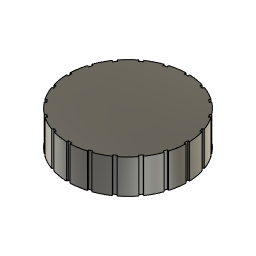
3DKNOB v3 (Autodesk Fusion 360 design; units mm, degrees)
Autodesk Fusion 360 part; units mm, degrees
sketch "Sketch1" plane through (0, 0, 0) normal (0, 0, 1) x (1, 0, 0)
  line L0 (0, 0) -> (124, 0)
  line L1 (124, 0) -> (124, 124)
  line L2 (124, 124) -> (0, 124)
  line L3 (0, 124) -> (0, 0)
  dimension "d1" = 124
  dimension "d2" = 124
  constraint horizontal L0
  constraint vertical L1
  constraint horizontal L2
  constraint vertical L3
  constraint coincident L0.start L3.end
  measures "d1" distance of L0.start L0.end
  measures "d2" distance of L0.start L2.end
sketch "Sketch3" plane through (0, 0, 5) normal (0, 0, 1) x (-1, 0, 0)
  line L0 (0, -124) -> (0, 0)
  line L1 (0, 0) -> (-124, 0)
  line L2 (-124, 0) -> (-124, -124)
  line L3 (-124, -124) -> (0, -124)
  line L4 (0, 0) -> (-124, 0)
  line L5 (-124, 0) -> (-124, -124)
  line L6 (-124, -124) -> (0, -124)
  line L7 (0, -124) -> (0, 0)
  line L8 (0, -124) -> (-124, -124)
  line L9 (-124, -124) -> (-124, 0)
  line L10 (-124, 0) -> (0, 0)
  line L11 (0, 0) -> (0, -124)
  line L12 (0, -124) -> (-7, -124)
  line L13 (-7, -124) -> (-7, -117)
  line L14 (-7, -117) -> (0, -117)
  line L15 (0, -117) -> (0, -124)
  line L16 (-7, -117) -> (-117, -117)
  line L17 (-117, -117) -> (-117, -7)
  line L18 (-117, -7) -> (-7, -7)
  line L19 (-7, -7) -> (-7, -117)
  line L20 (-7, -117) -> (-12, -117)
  line L21 (-12, -117) -> (-12, -112)
  line L22 (-12, -112) -> (-7, -112)
  line L23 (-7, -112) -> (-7, -117)
  line L24 (-12, -112) -> (-112, -112)
  line L25 (-112, -112) -> (-112, -12)
  line L26 (-112, -12) -> (-12, -12)
  line L27 (-12, -12) -> (-12, -112)
  dimension "d5" = 7
  dimension "d6" = 7
  dimension "d7" = 110
  dimension "d8" = 110
  dimension "d9" = 5
  dimension "d10" = 5
  dimension "d11" = 100
  dimension "d12" = 100
  constraint horizontal L4
  constraint vertical L5
  constraint horizontal L6
  constraint vertical L7
  constraint coincident L2.end L3.start
  constraint coincident L0.end L1.start
  constraint horizontal L8
  constraint vertical L9
  constraint horizontal L10
  constraint vertical L11
  constraint coincident L1.end L2.start
  constraint coincident L0.start L3.end
  constraint horizontal L12
  constraint vertical L13
  constraint horizontal L14
  constraint vertical L15
  constraint horizontal L16
  constraint vertical L17
  constraint horizontal L18
  constraint vertical L19
  constraint horizontal L20
  constraint vertical L21
  constraint horizontal L22
  constraint vertical L23
  constraint horizontal L24
  constraint vertical L25
  constraint horizontal L26
  constraint vertical L27
  measures "d5" distance of L0.start L12.end
  measures "d6" distance of L0.start L14.end
  measures "d7" distance of L13.end L16.end
  measures "d8" distance of L13.end L18.end
  measures "d9" distance of L13.end L20.end
  measures "d10" distance of L13.end L22.end
  measures "d11" distance of L21.end L24.end
  measures "d12" distance of L21.end L26.end
sketch "Sketch4" plane through (0, 12, 0) normal (0, -1, 0) x (1, 0, 0)
  line L0 (12, 5) -> (112, 5)
  line L1 (112, 5) -> (112, 10)
  line L2 (112, 10) -> (12, 10)
  line L3 (12, 10) -> (12, 5)
  line L4 (12, 5) -> (112, 5)
  line L5 (112, 5) -> (112, 75)
  line L6 (112, 75) -> (12, 75)
  line L7 (12, 75) -> (12, 5)
  line L8 (112, 5) -> (112, 22.5)
  line L9 (112, 22.5) -> (107, 22.5)
  line L10 (107, 22.5) -> (107, 17.5)
  line L11 (107, 17.5) -> (112, 17.5)
  line L12 (112, 17.5) -> (112, 22.5)
  line L13 (112, 22.5) -> (107, 22.5)
  line L14 (107, 22.5) -> (107, 27.5)
  line L15 (107, 27.5) -> (112, 27.5)
  line L16 (112, 27.5) -> (112, 22.5)
  line L17 (112, 75) -> (112, 57.5)
  line L18 (112, 57.5) -> (107, 57.5)
  line L19 (107, 57.5) -> (107, 62.5)
  line L20 (107, 62.5) -> (112, 62.5)
  line L21 (112, 62.5) -> (112, 57.5)
  line L22 (112, 57.5) -> (107, 57.5)
  line L23 (107, 57.5) -> (107, 52.5)
  line L24 (107, 52.5) -> (112, 52.5)
  line L25 (112, 52.5) -> (112, 57.5)
  line L26 (12, 75) -> (12, 57.5)
  line L27 (12, 57.5) -> (17, 57.5)
  line L28 (17, 57.5) -> (17, 62.5)
  line L29 (17, 62.5) -> (12, 62.5)
  line L30 (12, 62.5) -> (12, 57.5)
  line L31 (12, 57.5) -> (17, 57.5)
  line L32 (17, 57.5) -> (17, 52.5)
  line L33 (17, 52.5) -> (12, 52.5)
  line L34 (12, 52.5) -> (12, 57.5)
  line L35 (12, 5) -> (12, 22.5)
  line L36 (12, 22.5) -> (17, 22.5)
  line L37 (17, 22.5) -> (17, 27.5)
  line L38 (17, 27.5) -> (12, 27.5)
  line L39 (12, 27.5) -> (12, 22.5)
  line L40 (12, 22.5) -> (17, 22.5)
  line L41 (17, 22.5) -> (17, 17.5)
  line L42 (17, 17.5) -> (12, 17.5)
  line L43 (12, 17.5) -> (12, 22.5)
  line L44 (12, 62.5) -> (7, 62.5)
  line L45 (7, 62.5) -> (7, 52.5)
  line L46 (7, 52.5) -> (12, 52.5)
  line L47 (12, 52.5) -> (12, 62.5)
  line L48 (12, 27.5) -> (7, 27.5)
  line L49 (7, 27.5) -> (7, 17.5)
  line L50 (7, 17.5) -> (12, 17.5)
  line L51 (12, 17.5) -> (12, 27.5)
  line L52 (112, 62.5) -> (117, 62.5)
  line L53 (117, 62.5) -> (117, 52.5)
  line L54 (117, 52.5) -> (112, 52.5)
  line L55 (112, 52.5) -> (112, 62.5)
  line L56 (112, 27.5) -> (117, 27.5)
  line L57 (117, 27.5) -> (117, 17.5)
  line L58 (117, 17.5) -> (112, 17.5)
  line L59 (112, 17.5) -> (112, 27.5)
  dimension "d15" = 100
  dimension "d16" = 70
  dimension "d17" = 17.5
  dimension "d18" = 5
  dimension "d19" = 5
  dimension "d20" = 5
  dimension "d21" = 5
  dimension "d22" = 17.5
  dimension "d23" = 5
  dimension "d24" = 5
  dimension "d25" = 5
  dimension "d26" = 5
  dimension "d27" = 17.5
  dimension "d28" = 5
  dimension "d29" = 5
  dimension "d30" = 5
  dimension "d31" = 5
  dimension "d32" = 17.5
  dimension "d33" = 5
  dimension "d34" = 5
  dimension "d35" = 5
  dimension "d36" = 5
  dimension "d37" = 5
  dimension "d38" = 10
  dimension "d39" = 5
  dimension "d40" = 10
  dimension "d41" = 5
  dimension "d42" = 10
  dimension "d43" = 5
  dimension "d44" = 10
  constraint horizontal L4
  constraint vertical L5
  constraint horizontal L6
  constraint vertical L7
  constraint coincident L0.start L3.end
  constraint coincident L0.end L1.start
  constraint perpendicular L4 L8
  constraint horizontal L9
  constraint vertical L10
  constraint horizontal L11
  constraint vertical L12
  constraint horizontal L13
  constraint vertical L14
  constraint horizontal L15
  constraint vertical L16
  constraint perpendicular L6 L17
  constraint horizontal L18
  constraint vertical L19
  constraint horizontal L20
  constraint vertical L21
  constraint horizontal L22
  constraint vertical L23
  constraint horizontal L24
  constraint vertical L25
  constraint perpendicular L6 L26
  constraint horizontal L27
  constraint vertical L28
  constraint horizontal L29
  constraint vertical L30
  constraint horizontal L31
  constraint vertical L32
  constraint horizontal L33
  constraint vertical L34
  constraint perpendicular L4 L35
  constraint horizontal L36
  constraint vertical L37
  constraint horizontal L38
  constraint vertical L39
  constraint horizontal L40
  constraint vertical L41
  constraint horizontal L42
  constraint vertical L43
  constraint horizontal L44
  constraint vertical L45
  constraint horizontal L46
  constraint vertical L47
  constraint horizontal L48
  constraint vertical L49
  constraint horizontal L50
  constraint vertical L51
  constraint horizontal L52
  constraint vertical L53
  constraint horizontal L54
  constraint vertical L55
  constraint horizontal L56
  constraint vertical L57
  constraint horizontal L58
  constraint vertical L59
  measures "d15" distance of L0.start L0.end
  measures "d16" distance of L0.start L6.end
  measures "d17" distance of L0.end L8.end
  measures "d18" distance of L8.end L9.end
  measures "d19" distance of L8.end L11.end
  measures "d20" distance of L8.end L9.end
  measures "d21" distance of L8.end L15.end
  measures "d22" distance of L5.end L17.end
  measures "d23" distance of L17.end L18.end
  measures "d24" distance of L17.end L20.end
  measures "d25" distance of L17.end L18.end
  measures "d26" distance of L17.end L24.end
  measures "d27" distance of L6.end L26.end
  measures "d28" distance of L26.end L27.end
  measures "d29" distance of L26.end L29.end
  measures "d30" distance of L26.end L27.end
  measures "d31" distance of L26.end L33.end
  measures "d32" distance of L0.start L35.end
  measures "d33" distance of L35.end L36.end
  measures "d34" distance of L35.end L38.end
  measures "d35" distance of L35.end L36.end
  measures "d36" distance of L35.end L42.end
  measures "d37" distance of L29.end L44.end
  measures "d38" distance of L29.end L33.end
  measures "d39" distance of L38.end L48.end
  measures "d40" distance of L38.end L42.end
  measures "d41" distance of L20.end L52.end
  measures "d42" distance of L20.end L24.end
  measures "d43" distance of L15.end L56.end
  measures "d44" distance of L15.end L11.end
sketch "Sketch5" plane through (0, 112, 0) normal (0, 1, 0) x (-1, 0, 0)
  line L0 (-112, 5) -> (-12, 5)
  line L1 (-12, 5) -> (-12, 10)
  line L2 (-12, 10) -> (-112, 10)
  line L3 (-112, 10) -> (-112, 5)
  line L4 (-112, 5) -> (-12, 5)
  line L5 (-12, 5) -> (-12, 35)
  line L6 (-12, 35) -> (-112, 35)
  line L7 (-112, 35) -> (-112, 5)
  line L8 (-12, 35) -> (-12, 20)
  line L9 (-12, 20) -> (-7, 20)
  line L10 (-7, 20) -> (-7, 25)
  line L11 (-7, 25) -> (-12, 25)
  line L12 (-12, 25) -> (-12, 20)
  line L13 (-12, 20) -> (-7, 20)
  line L14 (-7, 20) -> (-7, 15)
  line L15 (-7, 15) -> (-12, 15)
  line L16 (-12, 15) -> (-12, 20)
  line L17 (-112, 20) -> (-117, 20)
  line L18 (-117, 20) -> (-117, 25)
  line L19 (-117, 25) -> (-112, 25)
  line L20 (-112, 25) -> (-112, 20)
  line L21 (-112, 20) -> (-117, 20)
  line L22 (-117, 20) -> (-117, 15)
  line L23 (-117, 15) -> (-112, 15)
  line L24 (-112, 15) -> (-112, 20)
  dimension "d47" = 100
  dimension "d48" = 30
  dimension "d49" = 15
  dimension "d50" = 5
  dimension "d51" = 5
  dimension "d52" = 5
  dimension "d53" = 5
  dimension "d54" = 5
  dimension "d55" = 5
  dimension "d56" = 5
  dimension "d57" = 5
  constraint horizontal L4
  constraint vertical L5
  constraint horizontal L6
  constraint vertical L7
  constraint coincident L0.start L3.end
  constraint perpendicular L6 L8
  constraint horizontal L9
  constraint vertical L10
  constraint horizontal L11
  constraint vertical L12
  constraint horizontal L13
  constraint vertical L14
  constraint horizontal L15
  constraint vertical L16
  constraint horizontal L17
  constraint vertical L18
  constraint horizontal L19
  constraint vertical L20
  constraint midpoint L7 L17.start
  constraint horizontal L21
  constraint vertical L22
  constraint horizontal L23
  constraint vertical L24
  measures "d47" distance of L0.start L0.end
  measures "d48" distance of L0.start L6.end
  measures "d49" distance of L5.end L8.end
  measures "d50" distance of L8.end L9.end
  measures "d51" distance of L8.end L11.end
  measures "d52" distance of L8.end L9.end
  measures "d53" distance of L8.end L15.end
  measures "d54" distance of L17.start L17.end
  measures "d55" distance of L17.start L19.end
  measures "d56" distance of L17.start L17.end
  measures "d57" distance of L17.start L23.end
sketch "Sketch6" plane through (12, 0, 0) normal (-1, 0, 0) x (0, -1, 0)
  line L0 (-112, 5) -> (-12, 5)
  line L1 (-12, 5) -> (-12, 10)
  line L2 (-12, 10) -> (-112, 10)
  line L3 (-112, 10) -> (-112, 5)
  line L4 (-117, 5) -> (-7, 5)
  line L5 (-7, 5) -> (-7, 35)
  line L6 (-7, 35) -> (-117, 35)
  line L7 (-117, 35) -> (-117, 5)
  line L8 (-117, 35) -> (-7, 75)
  line L9 (-7, 75) -> (-7, 35)
  line L10 (-7, 75) -> (-7, 62.5)
  line L11 (-7, 62.5) -> (-12, 62.5)
  line L12 (-12, 62.5) -> (-12, 52.5)
  line L13 (-12, 52.5) -> (-7, 52.5)
  line L14 (-7, 52.5) -> (-7, 62.5)
  line L15 (-7, 5) -> (-7, 17.5)
  line L16 (-7, 17.5) -> (-12, 17.5)
  line L17 (-12, 17.5) -> (-12, 27.5)
  line L18 (-12, 27.5) -> (-7, 27.5)
  line L19 (-7, 27.5) -> (-7, 17.5)
  line L20 (-117, 5) -> (-117, 15)
  line L21 (-117, 15) -> (-112, 15)
  line L22 (-112, 15) -> (-112, 25)
  line L23 (-112, 25) -> (-117, 25)
  line L24 (-117, 25) -> (-117, 15)
  dimension "d60" = 110
  dimension "d61" = 30
  dimension "d62" = 12.5
  dimension "d63" = 5
  dimension "d64" = 10
  dimension "d65" = 12.5
  dimension "d66" = 5
  dimension "d67" = 10
  dimension "d68" = 10
  dimension "d69" = 5
  dimension "d70" = 10
  constraint horizontal L4
  constraint vertical L5
  constraint horizontal L6
  constraint vertical L7
  constraint parallel L9 L10
  constraint vertical L12
  constraint perpendicular L11 L12
  constraint horizontal L13
  constraint parallel L12 L14
  constraint perpendicular L6 L15
  constraint vertical L17
  constraint perpendicular L16 L17
  constraint horizontal L18
  constraint parallel L17 L19
  constraint perpendicular L4 L20
  constraint horizontal L21
  constraint vertical L22
  constraint horizontal L23
  constraint vertical L24
  measures "d60" distance of L4.start L4.end
  measures "d61" distance of L4.start L6.end
  measures "d62" distance of L8.end L10.end
  measures "d63" distance of L10.end L11.end
  measures "d64" distance of L10.end L13.end
  measures "d65" distance of L4.end L15.end
  measures "d66" distance of L15.end L16.end
  measures "d67" distance of L15.end L18.end
  measures "d68" distance of L4.start L20.end
  measures "d69" distance of L20.end L21.end
  measures "d70" distance of L20.end L23.end
sketch "Sketch7" plane through (112, 0, 0) normal (1, 0, 0) x (0, 1, 0)
  line L0 (12, 5) -> (112, 5)
  line L1 (112, 5) -> (112, 10)
  line L2 (112, 10) -> (12, 10)
  line L3 (12, 10) -> (12, 5)
  line L4 (12, 5) -> (117, 5)
  line L5 (117, 5) -> (117, 35)
  line L6 (117, 35) -> (12, 35)
  line L7 (12, 35) -> (12, 5)
  line L8 (12, 5) -> (7, 5)
  line L9 (7, 5) -> (7, 35)
  line L10 (7, 35) -> (12, 35)
  line L11 (12, 35) -> (12, 5)
  line L12 (7, 35) -> (7, 75)
  line L13 (7, 75) -> (117, 35)
  line L14 (7, 75) -> (7, 62.5)
  line L15 (7, 62.5) -> (12, 62.5)
  line L16 (12, 62.5) -> (12, 52.5)
  line L17 (12, 52.5) -> (7, 52.5)
  line L18 (7, 52.5) -> (7, 62.5)
  line L19 (7, 5) -> (7, 17.5)
  line L20 (7, 17.5) -> (12, 17.5)
  line L21 (12, 17.5) -> (12, 27.5)
  line L22 (12, 27.5) -> (7, 27.5)
  line L23 (7, 27.5) -> (7, 17.5)
  line L24 (117, 20) -> (112, 20)
  line L25 (112, 20) -> (112, 25)
  line L26 (112, 25) -> (117, 25)
  line L27 (117, 25) -> (117, 20)
  line L28 (117, 20) -> (112, 20)
  line L29 (112, 20) -> (112, 15)
  line L30 (112, 15) -> (117, 15)
  line L31 (117, 15) -> (117, 20)
  dimension "d73" = 105
  dimension "d74" = 30
  dimension "d75" = 12.5
  dimension "d76" = 5
  dimension "d77" = 10
  dimension "d78" = 12.5
  dimension "d79" = 5
  dimension "d80" = 10
  dimension "d81" = 5
  dimension "d82" = 5
  dimension "d83" = 5
  dimension "d84" = 5
  constraint horizontal L4
  constraint vertical L5
  constraint horizontal L6
  constraint vertical L7
  constraint coincident L0.start L3.end
  constraint horizontal L8
  constraint vertical L9
  constraint horizontal L10
  constraint vertical L11
  constraint perpendicular L10 L12
  constraint perpendicular L6 L14
  constraint horizontal L15
  constraint vertical L16
  constraint horizontal L17
  constraint vertical L18
  constraint perpendicular L8 L19
  constraint horizontal L20
  constraint vertical L21
  constraint horizontal L22
  constraint vertical L23
  constraint horizontal L24
  constraint vertical L25
  constraint horizontal L26
  constraint vertical L27
  constraint midpoint L5 L24.start
  constraint horizontal L28
  constraint vertical L29
  constraint horizontal L30
  constraint vertical L31
  measures "d73" distance of L0.start L4.end
  measures "d74" distance of L0.start L6.end
  measures "d75" distance of L12.end L14.end
  measures "d76" distance of L14.end L15.end
  measures "d77" distance of L14.end L17.end
  measures "d78" distance of L8.end L19.end
  measures "d79" distance of L19.end L20.end
  measures "d80" distance of L19.end L22.end
  measures "d81" distance of L24.start L24.end
  measures "d82" distance of L24.start L26.end
  measures "d83" distance of L24.start L24.end
  measures "d84" distance of L24.start L30.end
sketch "Sketch8" plane through (112, 0, 0) normal (1, 0, 0) x (0, 1, 0)
  line L0 (12, 62.5) -> (12, 75)
  line L1 (12, 75) -> (7, 75)
  line L2 (7, 75) -> (7, 62.5)
  line L3 (7, 62.5) -> (12, 62.5)
  line L4 (12, 75) -> (12, 73.2)
  line L5 (12, 75) -> (7, 75)
  line L6 (7, 75) -> (12, 73.2)
  constraint coincident L0.end L1.start
  constraint coincident L0 L4.end
  constraint perpendicular L1 L4
  constraint coincident L1.end L2.start
sketch "Sketch9" plane through (0, 24.9051, 68.4891) normal (0, 0.341743, 0.939793) x (-1, 0, 0)
  line L0 (-12, 19.0522) -> (-12, -97.9948)
  line L1 (-12, -97.9948) -> (-7, -97.9948)
  line L2 (-7, -97.9948) -> (-7, 19.0522)
  line L3 (-7, 19.0522) -> (-12, 19.0522)
  line L4 (-112, 13) -> (-12, 13)
  line L5 (-12, 13) -> (-12, -93.0081)
  line L6 (-12, -93.0081) -> (-112, -93.0081)
  line L7 (-112, -93.0081) -> (-112, 13)
  constraint horizontal L4
  constraint vertical L5
  constraint horizontal L6
  constraint vertical L7
  constraint coincident L0 L5.end
sketch "Sketch10" plane through (0, 24.9051, 68.4891) normal (0, 0.341743, 0.939793) x (-1, 0, 0)
  line L0 (-112, -93.0081) -> (-12, -93.0081)
  line L1 (-12, -93.0081) -> (-12, 13)
  line L2 (-12, 13) -> (-112, 13)
  line L3 (-112, 13) -> (-112, -93.0081)
  line L4 (-117, -98) -> (-7, -98)
  line L5 (-7, -98) -> (-7, 19.05)
  line L6 (-7, 19.05) -> (-117, 19.05)
  line L7 (-117, 19.05) -> (-117, -98)
  constraint horizontal L4
  constraint vertical L5
  constraint horizontal L6
  constraint vertical L7
sketch "Sketch11" plane through (117, 0, 0) normal (1, 0, 0) x (0, 1, 0)
  line L0 (7.002, 74.9993) -> (117.0049, 34.9982)
  line L1 (117.0049, 34.9982) -> (118.7136, 39.6972)
  line L2 (118.7136, 39.6972) -> (8.7108, 79.6982)
  line L3 (8.7108, 79.6982) -> (7.002, 74.9993)
  line L4 (117.0049, 34.9982) -> (117.0049, 40.3185)
  line L5 (118.7136, 39.6972) -> (117.0049, 34.9982)
  line L6 (118.7136, 39.6972) -> (117.0049, 40.3185)
  constraint coincident L0.end L1.start
  constraint coincident L2 L4.end
  constraint vertical L4
  constraint coincident L1.end L2.start
sketch "Sketch14" plane through (0, 26.6138, 73.188) normal (0, 0.341743, 0.939793) x (-1, 0, 0)
  line L0 (-117, -96.1818) -> (-7, -96.1818)
  line L1 (-7, -96.1818) -> (-7, 19.05)
  line L2 (-7, 19.05) -> (-117, 19.05)
  line L3 (-117, 19.05) -> (-117, -96.1818)
  circle A0 centre (-62, -38.5659) radius 35
  line L4 (-62, -38.5659) -> (-62, -3.5659)
  line L5 (-62, -3.5659) -> (-61, -3.5659)
  line L6 (-61, -3.5659) -> (-61, -4.5659)
  line L7 (-61, -4.5659) -> (-62, -4.5659)
  line L8 (-62, -4.5659) -> (-62, -3.5659)
  line L9 (-62, -3.5659) -> (-63, -3.5659)
  line L10 (-63, -3.5659) -> (-63, -4.5659)
  line L11 (-63, -4.5659) -> (-62, -4.5659)
  line L12 (-62, -4.5659) -> (-62, -3.5659)
  dimension "d105" = 70
  dimension "d106" = 1
  dimension "d107" = 1
  dimension "d108" = 1
  constraint coincident A0.centre L4.start
  constraint coincident A0 L4.end
  constraint vertical L4
  constraint horizontal L5
  constraint vertical L6
  constraint horizontal L7
  constraint vertical L8
  constraint horizontal L9
  constraint vertical L10
  constraint horizontal L11
  constraint vertical L12
  measures "d105" diameter of A0
  measures "d106" distance of L4.end L5.end
  measures "d107" distance of L4.end L7.end
  measures "d108" distance of L4.end L7.end
extrude "Extrude12" add sketch "Sketch14" along normal blind 20 contours A0 L6 L7 L10 L11
pattern_circular "C-Pattern1" count 20 over 360 about axis through (62, 69.6927, 78.8043) along (0, 0.341743, 0.939793) of 3 faces at (62.3333, 33.1831, 77.8929) (63, 34.8438, 84.3828) (61, 32.8743, 78.0052)
sketch "Sketch15" plane through (0, 26.6138, 73.188) normal (0, -0.341743, -0.939793) x (1, 0, 0)
  line L0 (52.1399, -4.9835) -> (52.4445, -5.921)
  line L1 (52.4445, -5.921) -> (50.5424, -6.539)
  line L2 (50.5424, -6.539) -> (50.2378, -5.6015)
  arc A0 (50.2378, -5.6015) -> (42.2449, -9.6741) centre (62, -38.5659) ccw
  line L3 (42.2449, -9.6741) -> (42.8243, -10.4715)
  line L4 (42.8243, -10.4715) -> (41.2063, -11.6471)
  line L5 (41.2063, -11.6471) -> (40.6269, -10.8497)
  arc A1 (40.6269, -10.8497) -> (34.2838, -17.1928) centre (62, -38.5659) ccw
  line L6 (34.2838, -17.1928) -> (35.0812, -17.7722)
  line L7 (35.0812, -17.7722) -> (33.9056, -19.3902)
  line L8 (33.9056, -19.3902) -> (33.1082, -18.8108)
  arc A2 (33.1082, -18.8108) -> (29.0356, -26.8037) centre (62, -38.5659) ccw
  line L9 (29.0356, -26.8037) -> (29.9731, -27.1083)
  line L10 (29.9731, -27.1083) -> (29.3551, -29.0104)
  line L11 (29.3551, -29.0104) -> (28.4176, -28.7058)
  arc A3 (28.4176, -28.7058) -> (27.0143, -37.5659) centre (62, -38.5659) ccw
  line L12 (27.0143, -37.5659) -> (28, -37.5659)
  line L13 (28, -37.5659) -> (28, -39.5659)
  line L14 (28, -39.5659) -> (27.0143, -39.5659)
  arc A4 (27.0143, -39.5659) -> (28.4176, -48.426) centre (62, -38.5659) ccw
  line L15 (28.4176, -48.426) -> (29.3551, -48.1214)
  line L16 (29.3551, -48.1214) -> (29.9731, -50.0235)
  line L17 (29.9731, -50.0235) -> (29.0356, -50.3281)
  arc A5 (29.0356, -50.3281) -> (33.1082, -58.321) centre (62, -38.5659) ccw
  line L18 (33.1082, -58.321) -> (33.9056, -57.7416)
  line L19 (33.9056, -57.7416) -> (35.0812, -59.3596)
  line L20 (35.0812, -59.3596) -> (34.2838, -59.939)
  arc A6 (34.2838, -59.939) -> (40.6269, -66.2822) centre (62, -38.5659) ccw
  line L21 (40.6269, -66.2822) -> (41.2063, -65.4847)
  line L22 (41.2063, -65.4847) -> (42.8243, -66.6603)
  line L23 (42.8243, -66.6603) -> (42.2449, -67.4577)
  arc A7 (42.2449, -67.4577) -> (50.2378, -71.5303) centre (62, -38.5659) ccw
  line L24 (50.2378, -71.5303) -> (50.5424, -70.5928)
  line L25 (50.5424, -70.5928) -> (52.4445, -71.2108)
  line L26 (52.4445, -71.2108) -> (52.1399, -72.1483)
  arc A8 (52.1399, -72.1483) -> (61, -73.5516) centre (62, -38.5659) ccw
  line L27 (61, -73.5516) -> (61, -72.5659)
  line L28 (61, -72.5659) -> (63, -72.5659)
  line L29 (63, -72.5659) -> (63, -73.5516)
  arc A9 (63, -73.5516) -> (71.8601, -72.1483) centre (62, -38.5659) ccw
  line L30 (71.8601, -72.1483) -> (71.5555, -71.2108)
  line L31 (71.5555, -71.2108) -> (73.4576, -70.5928)
  line L32 (73.4576, -70.5928) -> (73.7622, -71.5303)
  arc A10 (73.7622, -71.5303) -> (81.7551, -67.4577) centre (62, -38.5659) ccw
  line L33 (81.7551, -67.4577) -> (81.1757, -66.6603)
  line L34 (81.1757, -66.6603) -> (82.7937, -65.4847)
  line L35 (82.7937, -65.4847) -> (83.3731, -66.2822)
  arc A11 (83.3731, -66.2822) -> (89.7163, -59.939) centre (62, -38.5659) ccw
  line L36 (89.7163, -59.939) -> (88.9188, -59.3596)
  line L37 (88.9188, -59.3596) -> (90.0944, -57.7416)
  line L38 (90.0944, -57.7416) -> (90.8918, -58.321)
  arc A12 (90.8918, -58.321) -> (94.9644, -50.3281) centre (62, -38.5659) ccw
  line L39 (94.9644, -50.3281) -> (94.0269, -50.0235)
  line L40 (94.0269, -50.0235) -> (94.6449, -48.1214)
  line L41 (94.6449, -48.1214) -> (95.5824, -48.426)
  arc A13 (95.5824, -48.426) -> (96.9857, -39.5659) centre (62, -38.5659) ccw
  line L42 (96.9857, -39.5659) -> (96, -39.5659)
  line L43 (96, -39.5659) -> (96, -37.5659)
  line L44 (96, -37.5659) -> (96.9857, -37.5659)
  arc A14 (96.9857, -37.5659) -> (95.5824, -28.7058) centre (62, -38.5659) ccw
  line L45 (95.5824, -28.7058) -> (94.6449, -29.0104)
  line L46 (94.6449, -29.0104) -> (94.0269, -27.1083)
  line L47 (94.0269, -27.1083) -> (94.9644, -26.8037)
  arc A15 (94.9644, -26.8037) -> (90.8918, -18.8108) centre (62, -38.5659) ccw
  line L48 (90.8918, -18.8108) -> (90.0944, -19.3902)
  line L49 (90.0944, -19.3902) -> (88.9188, -17.7722)
  line L50 (88.9188, -17.7722) -> (89.7163, -17.1928)
  arc A16 (89.7163, -17.1928) -> (83.3731, -10.8497) centre (62, -38.5659) ccw
  line L51 (83.3731, -10.8497) -> (82.7937, -11.6471)
  line L52 (82.7937, -11.6471) -> (81.1757, -10.4715)
  line L53 (81.1757, -10.4715) -> (81.7551, -9.6741)
  arc A17 (81.7551, -9.6741) -> (73.7622, -5.6015) centre (62, -38.5659) ccw
  line L54 (73.7622, -5.6015) -> (73.4576, -6.539)
  line L55 (73.4576, -6.539) -> (71.5555, -5.921)
  line L56 (71.5555, -5.921) -> (71.8601, -4.9835)
  arc A18 (71.8601, -4.9835) -> (63, -3.5802) centre (62, -38.5659) ccw
  line L57 (63, -3.5802) -> (63, -4.5659)
  line L58 (63, -4.5659) -> (61, -4.5659)
  line L59 (61, -4.5659) -> (61, -3.5802)
  arc A19 (61, -3.5802) -> (52.1399, -4.9835) centre (62, -38.5659) ccw
  circle A20 centre (62, -38.5659) radius 3
  line L60 (62, -38.5659) -> (62, -38.1159)
  line L61 (62, -38.5659) -> (62, -39.0159)
  line L62 (62, -38.1159) -> (64.9661, -38.1159)
  line L63 (62, -39.0159) -> (64.9661, -39.0159)
  line L64 (62, -38.1159) -> (59.0339, -38.1159)
  line L65 (62, -39.0159) -> (59.0339, -39.0159)
  dimension "d115" = 6
  dimension "d116" = 0.45
  dimension "d117" = 0.45
  constraint concentric A0 A20
  constraint coincident A0.centre A1.centre
  constraint vertical L60
  constraint parallel L60 L61
  constraint coincident A20 L62.end
  constraint perpendicular L60 L62
  constraint coincident A20 L63.end
  constraint perpendicular L61 L63
  constraint coincident A20 L64.end
  constraint perpendicular L60 L64
  constraint coincident A20 L65.end
  constraint perpendicular L61 L65
  measures "d115" diameter of A20
  measures "d116" distance of A0.centre L60.end
  measures "d117" distance of A0.centre L61.end
extrude "Extrude13" cut sketch "Sketch15" against normal blind 10 contours A20 L62 L64 | A20 L63 L65
sketch "Sketch16" plane through (0, 24.9051, 68.4891) normal (0, -0.341743, -0.939793) x (1, 0, 0)
  line L0 (117, -98) -> (117, 19.05)
  line L1 (117, 19.05) -> (7, 19.05)
  line L2 (7, 19.05) -> (7, -98)
  line L3 (7, -98) -> (117, -98)
  circle A0 centre (62, -39.475) radius 4
  dimension "d120" = 8
  measures "d120" diameter of A0
sketch "Sketch17" plane through (0, 24.9051, 68.4891) normal (0, 0.341743, 0.939793) x (-1, 0, 0)
  line L0 (-112, -93.0081) -> (-12, -93.0081)
  line L1 (-12, -93.0081) -> (-12, 13)
  line L2 (-12, 13) -> (-112, 13)
  line L3 (-112, 13) -> (-112, -93.0081)
  circle A0 centre (-62, -39.474) radius 4
  dimension "d123" = 8
  measures "d123" diameter of A0
sketch "Sketch18" plane through (12, 0, 0) normal (-1, 0, 0) x (0, -1, 0)
  line L0 (-12.6878, 72.9317) -> (-112.3135, 36.7042)
  line L1 (-112.3135, 36.7042) -> (-110.6048, 32.0052)
  line L2 (-110.6048, 32.0052) -> (-10.9791, 68.2327)
  line L3 (-10.9791, 68.2327) -> (-12.6878, 72.9317)
  line L4 (-12.6878, 72.9317) -> (-12.6878, 67.6114)
  line L5 (-12.6878, 67.6114) -> (-10.9791, 68.2327)
  line L6 (-12.6878, 72.9317) -> (-10.9791, 68.2327)
  constraint coincident L0.start L3.end
  constraint coincident L2 L4.end
  constraint vertical L4
  constraint coincident L2.end L3.start
sketch "Sketch19" plane through (0, 0, 0) normal (0, 0, 1) x (1, 0, 0)
  line L0 (0, 0) -> (126.9963, 0)
  line L1 (126.9963, 0) -> (126.9963, 102.615)
  line L2 (126.9963, 102.615) -> (0, 102.615)
  line L3 (0, 102.615) -> (0, 0)
  constraint horizontal L0
  constraint vertical L1
  constraint horizontal L2
  constraint vertical L3
  constraint coincident L0.start L3.end
move_body "Align1" bodies 1 to x (1, 0, 0) y (0, 0.939793, 0.341743) z (0, -0.341743, 0.939793) at (0, 24.2915, -67.8767)
